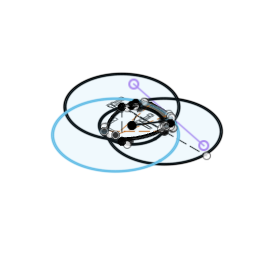
langer_schwede_v2 (Autodesk Fusion 360 design; units mm, degrees)
Autodesk Fusion 360 part; units mm, degrees
sketch "Sketch1" plane through (0, 0, 0) normal (0, 0, 1) x (1, 0, 0)
  circle A0 centre (0, 0) radius 85
  circle A1 centre (0, -62) radius 170
  circle A2 centre (0, 0) radius 89
  circle A3 centre (80, 42) radius 150
  circle A4 centre (-80, 42) radius 150
  circle A5 centre (-66, 80) radius 10
  circle A6 centre (-66, 80) radius 14
  circle A7 centre (80, 42) radius 154
  circle A8 centre (-80, 42) radius 154
  circle A9 centre (66, 80) radius 10
  circle A10 centre (66, 80) radius 14
  line L0 (0, 0) -> (-54.0969, 87.37) construction
  line L1 (0, 0) -> (54.0969, 87.37)
  line L2 (-56, 80) -> (-56, 98.5117)
  line L3 (-52, 80) -> (-52, 99.8518)
  circle A11 centre (0, -62) radius 166
  line L4 (56, 80) -> (56, 98.5117)
  line L5 (52, 80) -> (52, 99.8518)
  line L6 (52, 99.8518) -> (44.7466, 72.2686)
  line L7 (-80, 42) -> (33.1371, -71.1371) construction
  line L8 (-80, 42) -> (80, 42) construction
  circle A12 centre (33.1371, -71.1371) radius 10
  circle A13 centre (33.1371, -71.1371) radius 6
  line L9 (80, 42) -> (-33.1371, -71.1371) construction
  line L10 (80, 42) -> (240, 42) construction
  circle A14 centre (-33.1371, -71.1371) radius 10
  circle A15 centre (-33.1371, -71.1371) radius 6
  line L11 (-33.1371, -71.1371) -> (-47.2792, -56.9949)
  line L12 (-33.1371, -71.1371) -> (-13.1371, -71.1371) construction
  line L13 (33.1371, -71.1371) -> (47.2792, -56.9949)
  line L14 (33.1371, -71.1371) -> (53.1371, -71.1371) construction
  line L15 (-66, 80) -> (-66, 48.7192) construction
  line L16 (66, 80) -> (66, 44.8781) construction
  line L17 (66, 70) -> (86, 70) construction
  line L18 (66, 70) -> (72.4905, 63.5095) construction
  line L19 (66, 70) -> (75.1789, 70) construction
  line L20 (69.2452, 66.7548) -> (62.7188, 60.2283) construction
  circle A16 centre (65.982, 63.4915) radius 6.5085
  circle A17 centre (65.982, 63.4915) radius 2.5085
  circle A18 centre (0, 0) radius 86.6
  line L21 (-66, 70) -> (-72.4905, 63.5095) construction
  line L22 (-66, 70) -> (-56.8211, 70) construction
  line L23 (-69.2452, 66.7548) -> (-66, 63.5095) construction
  circle A19 centre (-66, 63.5095) radius 6.4905
  circle A20 centre (-66, 63.5095) radius 2.4905
  line L24 (50.4526, 100.2587) -> (43.1992, 72.6755)
  line L25 (-52, 99.8518) -> (-44.7466, 72.2686)
  line L26 (-50.4526, 100.2587) -> (-43.1992, 72.6755)
  line L27 (0, 108) -> (35.2, 108) construction
  line L28 (0, -62) -> (35.2, 108) construction
  line L29 (34.4689, 104.4689) -> (42.2819, 102.8512) construction
  line L30 (0, 108) -> (-35.2, 108) construction
  line L31 (-35.2, 108) -> (0, -62) construction
  line L32 (-34.4689, 104.4689) -> (-54.0534, 100.4138) construction
  line L33 (66, 66) -> (86, 66) construction
  line L34 (68.0676, 66) -> (69.9855, 44.0838) construction
  line L35 (69.9855, 44.0838) -> (73.9859, 44.0838) construction
  line L36 (-69.9855, 44.0838) -> (-73.9859, 44.0838)
  line L37 (69.9855, 44.0838) -> (-69.9855, 44.0838) construction
  dimension "d1" = 170
  dimension "d2" = 340
  dimension "d3" = 62
  dimension "d14" = 4
  dimension "d15" = 300
  dimension "d16" = 42
  dimension "d17" = 80
  dimension "d18" = 300
  dimension "d19" = 80
  dimension "d20" = 42
  dimension "d21" = 20
  dimension "d22" = 80
  dimension "d23" = 66
  dimension "d24" = 4
  dimension "d28" = 4
  dimension "d31" = 4
  dimension "d36" = 20
  dimension "d37" = 66
  dimension "d38" = 80
  dimension "d39" = 4
  dimension "d40" = -4
  dimension "d46" = 45
  dimension "d47" = 160
  dimension "d48" = 20
  dimension "d49" = 12
  dimension "d50" = 135
  dimension "d51" = 160
  dimension "d52" = 20
  dimension "d53" = 12
  dimension "d54" = 135
  dimension "d55" = 20
  dimension "d56" = 45
  dimension "d57" = 20
  dimension "d61" = 45
  dimension "d62" = 135
  dimension "d63" = -4
  dimension "d64" = 1.6
  dimension "d68" = 135
  dimension "d69" = 45
  dimension "d70" = -4
  dimension "d71" = 1.6
  dimension "d73" = -1.6
  dimension "d78" = 35.2
  dimension "d86" = 35.2
  dimension "d87" = 20
  dimension "d95" = 20
  dimension "d96" = 22
  constraint coincident A0.centre A2.centre
  constraint coincident A6 L0.end
  constraint tangent A6 L0
  constraint coincident A10 L1.end
  constraint tangent A10 L1
  constraint coincident A5 L2.start
  constraint coincident A1 L2.end
  constraint tangent A5 L2
  constraint vertical L2
  constraint coincident A6 L3.start
  constraint coincident A1 L3.end
  constraint tangent A6 L3
  constraint parallel L2 L3
  constraint coincident A9 L4.start
  constraint coincident A1 L4.end
  constraint tangent A9 L4
  constraint vertical L4
  constraint coincident A10 L5.start
  constraint coincident A1 L5.end
  constraint tangent A10 L5
  constraint parallel L4 L5
  constraint coincident L1 L6.end
  constraint coincident A0 L6.end
  constraint horizontal L8
  constraint coincident A4.centre A8.centre
  constraint coincident L7.end A12.centre
  constraint concentric A12 A13
  constraint horizontal L10
  constraint coincident L9.end A14.centre
  constraint concentric A14 A15
  constraint horizontal L12
  constraint horizontal L14
  constraint coincident A5.centre A6.centre
  constraint vertical L15
  constraint coincident A9.centre A10.centre
  constraint vertical L16
  constraint horizontal L17
  constraint coincident L16 L17.start
  constraint coincident A9 L17.start
  constraint horizontal L19
  constraint coincident A8 L18.end
  constraint midpoint L18 L20.start
  constraint midpoint L20 A16.centre
  constraint coincident L17.start A16
  constraint horizontal L22
  constraint coincident A5 L21.start
  constraint coincident L15 L21.start
  constraint coincident A7 L21.end
  constraint midpoint L21 L23.start
  constraint coincident L15 L23.end
  constraint coincident L23.end A19.centre
  constraint coincident L21.start A19
  constraint coincident A0 L25.end
  constraint coincident L0 L25.end
  constraint coincident A1 L27.start
  constraint horizontal L27
  constraint coincident A1.centre A11.centre
  constraint coincident L28 L29.start
  constraint coincident A1 L29.start
  constraint tangent A1 L29
  constraint horizontal L30
  constraint coincident A1 L32.start
  constraint coincident L31 L32.start
  constraint tangent A1 L32
  constraint coincident L16 L33.start
  constraint coincident A10 L33.start
  constraint perpendicular L16 L33
  constraint coincident A4 L34.start
  constraint coincident L33 L34.start
  constraint coincident A4 L34.end
  constraint coincident A8 L35.end
  constraint horizontal L35
  constraint coincident A3 L36.start
  constraint coincident A7 L36.end
  constraint horizontal L36
  constraint horizontal L37
  constraint coincident L36 L37.end
  measures "d1" diameter of A0
  measures "d2" diameter of A1
  measures "d3" distance of A0.centre A1.centre
  measures "d15" diameter of A3
  measures "d16" vertical distance of A0.centre A3.centre
  measures "d17" horizontal distance of A0.centre A3.centre
  measures "d18" diameter of A4
  measures "d19" horizontal distance of A0.centre A4.centre
  measures "d20" vertical distance of A0.centre A4.centre
  measures "d21" diameter of A5
  measures "d22" vertical distance of A0.centre A5.centre
  measures "d23" horizontal distance of A0.centre A5.centre
  measures "d36" diameter of A9
  measures "d37" horizontal distance of A0.centre A9.centre
  measures "d38" vertical distance of A0.centre A9.centre
  measures "d46" angle of L7 L8
  measures "d47" distance of A4.centre L7.end
  measures "d48" diameter of A12
  measures "d49" diameter of A13
  measures "d50" angle of L9 L10
  measures "d51" distance of A3.centre L9.end
  measures "d52" diameter of A14
  measures "d53" diameter of A15
  measures "d54" angle of L11 L12
  measures "d55" distance of L9.end L11.end
  measures "d56" angle of L13 L14
  measures "d57" distance of L7.end L13.end
  measures "d61" angle of L18 L19
  measures "d62" angle of L19 L20
  measures "d68" angle of L21 L22
  measures "d69" angle of L22 L23
  measures "d78" distance of L27.start L27.end
  measures "d86" distance of L27.start L30.end
  measures "d87" distance of L32.start L32.end
  measures "d95" distance of L33.start L33.end
  measures "d96" distance of L34.start L34.end
extrude "Extrude1" add sketch "Sketch1" along normal blind 5 contours A0 A4 A8 A12 | A0 A4 A8 A18 | A0 A12 A18 | A0 A8 A12 A13 L13 | A8 A12 | A12 A18 | A0 L6 A18 L24 | A2 A4 A8 A18 | A0 A18 L24 L26 | A2 L6 A18 L24 | A2 A4 A8 A16 | A0 A18 L25 L26 | A2 A11 L6 L24 | A4 A8 A10 A16 A17 | A0 A3 A7 A14 L36 | A7 A14 | A2 A18 L25 L26 | A10 L1 A11 L4 L5 | A10 L1 L5 | A11 L5 L6 | A1 A11 L6 L25 | A4 A17 | A0 A3 L36 | A0 A3 A7 A18 L36 | A2 A11 L25 L26 | A4 A10 A16 | A9 A10 L4 A16 | A1 A11 L4 L5 | A4 A10 A17 | A0 A7 L36 | A0 A7 A14 A15 L11 | A0 A14 A18 | A4 A10 A16 | A2 A3 A7 A18 | A1 L2 L3 A11 | L3 A11 L25 | A14 A18 | A2 A3 A7 A19 | A6 L2 L3 A11 | A3 A6 A7 A19 A20 | A5 A6 L2 A19 | A3 A6 A19 | A3 A6 A20 | A3 A6 A19 picked at (68.4239, 63.833)
extrude "Extrude2" add sketch "Sketch1" along normal blind 0.75 contours A2 A18 L24 L26 | A2 A11 L24 L26
fillet "Fillet1" radius 4 6 edges at (56, 98.5117, 2.5) (-56, 98.5117, 2.5) (-49.4543, 96.4622, 2.875) (-44.7466, 72.2686, 2.5) (44.7466, 72.2686, 2.5) (49.4543, 96.4622, 2.875)
fillet "Fillet2" radius 1 4 edges at (50.9812, 95.9776, 2.5) (52, 95.6452, 2.5) (-52, 95.6452, 2.5) (-50.9812, 95.9776, 2.5)
fillet "Fillet3" radius 2 6 edges at (43.7423, 74.7407, 2.875) (-43.7423, 74.7407, 2.875) (-37.3797, -66.8944, 2.5) (-40.2082, -64.066, 2.5) (37.3797, -66.8944, 2.5) (40.2082, -64.066, 2.5)
ref_plane "WorkPlane1" through (38.3754, 103.66, 0) normal (-0.202758, -0.979229, 0) x (0.979229, -0.202758, 0)
sketch "Sketch4" plane through (38.3754, 103.66, 0) normal (-0.202758, -0.979229, 0) x (0.979229, -0.202758, 0)
  circle A0 centre (-3.9894, 2.5) radius 2.5
  line L0 (166.0106, 0) -> (-173.9894, 0)
  dimension "d80" = 5
  dimension "d81" = 2.5
  measures "d80" diameter of A0
  measures "d81" distance of A0.centre L0
extrude "Extrude3" add sketch "Sketch4" along normal blind 1 and the other way blind 4
ref_plane "WorkPlane2" through (-44.2611, 102.4413, 0) normal (-0.202758, 0.979229, 0) x (-0.979229, -0.202758, 0)
sketch "Sketch5" plane through (-44.2611, 102.4413, 0) normal (-0.202758, 0.979229, 0) x (-0.979229, -0.202758, 0)
  circle A0 centre (-10.0017, 2.5) radius 2.5
  line L0 (201.2515, 0) -> (-106.7485, 0)
  dimension "d89" = 5
  dimension "d94" = 2.5
  measures "d89" diameter of A0
  measures "d94" distance of A0.centre L0
extrude "Extrude4" add sketch "Sketch5" along normal blind 4 and the other way blind 1
ref_plane "WorkPlane3" through (73.9859, 44.0838, 0) normal (0.999908, 0.013531, 0) x (-0.013531, 0.999908, 0)
sketch "Sketch6" plane through (73.9859, 44.0838, 0) normal (0.999908, 0.013531, 0) x (-0.013531, 0.999908, 0)
  circle A0 centre (0, 2.5) radius 2.5
  dimension "d97" = 5
  dimension "d98" = 2.5
  measures "d97" diameter of A0
  measures "d98" distance of origin A0.centre
extrude "Extrude5" add sketch "Sketch6" along normal blind 4 and the other way blind 1
ref_plane "WorkPlane4" through (-73.9859, 44.0838, 0) normal (-0.999908, 0.013531, 0) x (-0.013531, -0.999908, 0)
sketch "Sketch7" plane through (-73.9859, 44.0838, 0) normal (-0.999908, 0.013531, 0) x (-0.013531, -0.999908, 0)
  circle A0 centre (0, 2.5) radius 2.5
  dimension "d103" = 5
  dimension "d104" = 2.5
  measures "d103" diameter of A0
  measures "d104" distance of origin A0.centre
extrude "Extrude6" add sketch "Sketch7" along normal blind 4 and the other way blind 1
ref_plane "WorkPlane5" through (77.9855, 44.1379, 2.5) normal (0.999908, 0.013531, 0) x (-0.013531, 0.999908, 0)
sketch "Sketch8" plane through (77.9855, 44.1379, 2.5) normal (0.999908, 0.013531, 0) x (-0.013531, 0.999908, 0)
  circle A0 centre (0, 0) radius 2.5
  circle A1 centre (-2, 0) radius 2.5
  line L0 (-2, 2.5) -> (0, 2.5)
  line L1 (-2, -2.5) -> (0, -2.5)
  dimension "d110" = 5
  dimension "d111" = 5
  dimension "d112" = 2
  constraint coincident A0.centre origin
  constraint coincident A1 L0.start
  constraint coincident A0 L0.end
  constraint tangent A0 L0
  constraint horizontal L0
  constraint coincident A1 L1.start
  constraint coincident A0 L1.end
  constraint tangent A0 L1
  constraint horizontal L1
  measures "d110" diameter of A0
  measures "d111" diameter of A1
  measures "d112" distance of A0.centre A1.centre
extrude "Extrude7" add sketch "Sketch8" against normal blind 2
ref_plane "WorkPlane6" through (-77.9855, 44.1379, 2.5) normal (-0.999908, 0.013531, 0) x (-0.013531, -0.999908, 0)
sketch "Sketch9" plane through (-77.9855, 44.1379, 2.5) normal (-0.999908, 0.013531, 0) x (-0.013531, -0.999908, 0)
  circle A0 centre (0, 0) radius 2.5
  circle A1 centre (2, 0) radius 2.5
  line L0 (2, -2.5) -> (0, -2.5)
  line L1 (2, 2.5) -> (0, 2.5)
  dimension "d116" = 5
  dimension "d117" = 5
  dimension "d118" = 2
  constraint coincident A0.centre origin
  constraint coincident A1 L0.start
  constraint coincident A0 L0.end
  constraint tangent A0 L0
  constraint horizontal L0
  constraint coincident A1 L1.start
  constraint coincident A0 L1.end
  constraint tangent A0 L1
  constraint parallel L0 L1
  measures "d116" diameter of A0
  measures "d117" diameter of A1
  measures "d118" distance of A0.centre A1.centre
extrude "Extrude8" add sketch "Sketch9" against normal blind 2
